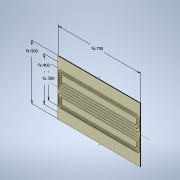
# Autodesk Inventor part: coil_layer_1R1
Saved by Autodesk Inventor 2021 (Build 250183000, 183)
## iProperties
Created: 2021-01-20
Part Number: coil_layer_1R1
Material: Generic
Document SubType Name: Modeling
Designer: phamv
Density: 1 g/cm^3
Appearance: Smooth - Ash
Author: phamv
Autodesk Inventor part; units mm, degrees
ref_plane "YZ Plane" through (0, 0, 0) normal (1, 0, 0) x (0, 1, 0)
ref_plane "XZ Plane" through (0, 0, 0) normal (0, 1, 0) x (-1, 0, 0)
ref_plane "XY Plane" through (0, 0, 0) normal (0, 0, 1) x (1, 0, 0)
sketch "layer_layout_sketch" plane through (0, 0, 0) normal (0, 0, 1) x (1, 0, 0)
  line L0 (-375, 250) -> (375, 250)
  line L1 (375, 250) -> (375, -250)
  line L2 (375, -250) -> (-375, -250)
  line L3 (-375, -250) -> (-375, 250)
  line L4 (0, 250) -> (0, -250) construction
  line L5 (-375, 200) -> (375, 200)
  line L6 (375, 200) -> (375, -200)
  line L7 (375, -200) -> (-375, -200)
  line L8 (-375, -200) -> (-375, 200)
  line L9 (0, 200) -> (0, -200) construction
  line L10 (-375, 150) -> (375, 150)
  line L11 (375, 150) -> (375, -150)
  line L12 (375, -150) -> (-375, -150)
  line L13 (-375, -150) -> (-375, 150)
  line L14 (0, 150) -> (0, -150) construction
  point P0 (0, 0)
  point P1 (0, 0)
  dimension "d116" = 500
  dimension "d117" = 750
  dimension "d122" = 400
  dimension "d123" = 300
  constraints: 30 end point, 9 midpoint, 6 parallel, 3 horizontal, 3 perpendicular, 2 collinear, 1 coincident, 1 vertical
  measures "d116" distance between parallel lines of L2 L0
  measures "d117" distance between parallel lines of L1 L3
  measures "d122" distance between parallel lines of L7 L5
  measures "d123" distance between parallel lines of L12 L10
sketch "coil_layer_sketch_lower" plane through (0, 0, 0) normal (0, 0, 1) x (1, 0, 0)
  line L0 (0, -9.3) -> (351.5, -9.3)
  line L1 (370, -27.8) -> (370, -131.5)
  line L2 (351.5, -150) -> (-351.5, -150)
  line L3 (-370, -131.5) -> (-370, -50.9)
  line L4 (0, -9.3) -> (0, -13.8)
  line L5 (0, -13.8) -> (350.5, -13.8)
  line L6 (365.5, -28.8) -> (365.5, -130.5)
  line L7 (350.5, -145.5) -> (-350.5, -145.5)
  line L8 (-351.5, -32.4) -> (338.75, -32.4)
  line L9 (357.25, -50.9) -> (357.25, -118.75)
  line L10 (338.75, -137.25) -> (-338.75, -137.25)
  line L11 (-365.5, -130.5) -> (-365.5, -51.9)
  line L12 (-350.5, -36.9) -> (337.75, -36.9)
  line L13 (352.75, -51.9) -> (352.75, -117.75)
  line L14 (337.75, -132.75) -> (-337.75, -132.75)
  line L15 (-352.75, -117.75) -> (-352.75, -75)
  line L16 (-357.25, -118.75) -> (-357.25, -74)
  line L17 (-338.75, -55.5) -> (326, -55.5)
  line L18 (344.5, -74) -> (344.5, -106)
  line L19 (-337.75, -60) -> (325, -60)
  line L20 (340, -75) -> (340, -105)
  line L21 (-523.3641, 0) -> (523.3641, 0) projected
  line L22 (325, -120) -> (-325, -120)
  line L23 (326, -124.5) -> (-326, -124.5)
  line L24 (-344.5, -106) -> (-344.5, -71.7563)
  line L25 (-344.5, -71.7563) -> (-340, -71.7563)
  line L26 (-340, -71.7563) -> (-340, -105)
  arc A0 (370, -27.8) -> (351.5, -9.3) centre (351.5, -27.8) ccw
  arc A1 (357.25, -50.9) -> (338.75, -32.4) centre (338.75, -50.9) ccw
  arc A2 (344.5, -74) -> (326, -55.5) centre (326, -74) ccw
  arc A3 (326, -124.5) -> (344.5, -106) centre (326, -106) ccw
  arc A4 (338.75, -137.25) -> (357.25, -118.75) centre (338.75, -118.75) ccw
  arc A5 (351.5, -150) -> (370, -131.5) centre (351.5, -131.5) ccw
  arc A6 (-370, -131.5) -> (-351.5, -150) centre (-351.5, -131.5) ccw
  arc A7 (-357.25, -118.75) -> (-338.75, -137.25) centre (-338.75, -118.75) ccw
  arc A8 (-344.5, -106) -> (-326, -124.5) centre (-326, -106) ccw
  arc A9 (-351.5, -32.4) -> (-370, -50.9) centre (-351.5, -50.9) ccw
  arc A10 (-338.75, -55.5) -> (-357.25, -74) centre (-338.75, -74) ccw
  arc A11 (-350.5, -36.9) -> (-365.5, -51.9) centre (-350.5, -51.9) ccw
  arc A12 (-337.75, -60) -> (-352.75, -75) centre (-337.75, -75) ccw
  arc A13 (-365.5, -130.5) -> (-350.5, -145.5) centre (-350.5, -130.5) ccw
  arc A14 (-352.75, -117.75) -> (-337.75, -132.75) centre (-337.75, -117.75) ccw
  arc A15 (-340, -105) -> (-325, -120) centre (-325, -105) ccw
  arc A16 (325, -120) -> (340, -105) centre (325, -105) ccw
  arc A17 (337.75, -132.75) -> (352.75, -117.75) centre (337.75, -117.75) ccw
  arc A18 (350.5, -145.5) -> (365.5, -130.5) centre (350.5, -130.5) ccw
  arc A19 (352.75, -51.9) -> (337.75, -36.9) centre (337.75, -51.9) ccw
  arc A20 (365.5, -28.8) -> (350.5, -13.8) centre (350.5, -28.8) ccw
  arc A21 (340, -75) -> (325, -60) centre (325, -75) ccw
  point P0 (0, 0)
  point P1 (0, 0)
  point P2 (368.0934, -60)
  point P3 (370, -61.9066)
  point P4 (0, -150)
  dimension "d1" = 4.5
  dimension "d2" = 4.5
  dimension "d3" = 4.5
  dimension "d4" = 9.3
  dimension "d5" = 740
  dimension "d6" = 370
  dimension "d7" = 4.5
  dimension "d8" = 4.5
  dimension "d9" = 8.25
  dimension "d10" = 4.5
  dimension "d11" = 18.6
  dimension "d12" = 4.5
  dimension "d13" = 8.25
  dimension "d14" = 4.5
  dimension "d15" = 4.5
  dimension "d16" = 4.5
  dimension "d17" = 8.25
  dimension "d19" = 18.6
  dimension "d20" = 8.25
  dimension "d82" = 150
  dimension "d88" = 4.5
  dimension "d89" = 8.25
  dimension "d96" = 4.5
  dimension "d97" = 8.25
  dimension "d98" = 18.5
  dimension "d99" = 15
  dimension "d109" = 15
  constraints: 52 end point, 44 point on circle, 44 tangent, 22 centre point, 19 equal radius, 15 perpendicular, 4 horizontal, 4 vertical, 3 parallel, 1 coincident, 1 midpoint
  measures "d1" distance between parallel lines of L5 L0
  measures "d2" distance between parallel lines of L6 L1
  measures "d3" distance between parallel lines of L2 L7
  measures "d4" distance from line of L21 L0.start
  measures "d5" distance between parallel lines of L3 L1
  measures "d6" distance from line of point (0, 0) L1
  measures "d7" distance between parallel lines of L3 L11
  measures "d8" distance between parallel lines of L13 L9
  measures "d9" distance between parallel lines of L9 L6
  measures "d10" distance between parallel lines of L8 L12
  measures "d11" distance between parallel lines of L8 L5
  measures "d12" distance between parallel lines of L10 L14
  measures "d13" distance between parallel lines of L7 L10
  measures "d14" distance between parallel lines of L16 L15
  measures "d15" distance between parallel lines of L17 L19
  measures "d16" distance between parallel lines of L20 L18
  measures "d17" distance between parallel lines of L18 L13
  measures "d19" distance between parallel lines of L17 L12
  measures "d20" distance between parallel lines of L11 L16
  measures "d82" distance between parallel lines of L2 L21
  measures "d88" distance between parallel lines of L23 L22
  measures "d89" distance between parallel lines of L14 L23
  measures "d96" distance between parallel lines of L24 L26
  measures "d97" distance between parallel lines of L15 L24
  measures "d98" radius of A0
  measures "d99" radius of A11
  measures "d109" radius of A21
sketch "coil_layer_sketch_upper" plane through (0, 0, 0) normal (0, 0, 1) x (1, 0, 0)
  line L0 (0, -13.8) -> (-351.5, -13.8)
  line L1 (-370, 4.7) -> (-370, 131.5)
  line L2 (-351.5, 150) -> (351.5, 150)
  line L3 (370, 131.5) -> (370, 27.8)
  line L4 (0, -9.3) -> (-350.5, -9.3)
  line L5 (-365.5, 5.7) -> (-365.5, 130.5)
  line L6 (-350.5, 145.5) -> (350.5, 145.5)
  line L7 (365.5, 130.5) -> (365.5, 28.8)
  line L8 (350.5, 13.8) -> (-337.75, 13.8)
  line L9 (-352.75, 28.8) -> (-352.75, 117.75)
  line L10 (351.5, 9.3) -> (-338.75, 9.3)
  line L11 (-357.25, 27.8) -> (-357.25, 118.75)
  line L12 (-337.75, 132.75) -> (337.75, 132.75)
  line L13 (-338.75, 137.25) -> (338.75, 137.25)
  line L14 (352.75, 117.75) -> (352.75, 51.9)
  line L15 (337.75, 36.9) -> (-325, 36.9)
  line L16 (357.25, 118.75) -> (357.25, 50.9)
  line L17 (338.75, 32.4) -> (-326, 32.4)
  line L18 (-340, 51.9) -> (-340, 105)
  line L19 (-325, 120) -> (325, 120)
  line L20 (340, 105) -> (340, 75)
  line L21 (325, 60) -> (-331.75, 60)
  line L22 (-344.5, 50.9) -> (-344.5, 106)
  line L23 (-326, 124.5) -> (326, 124.5)
  line L24 (344.5, 106) -> (344.5, 74)
  line L25 (326, 55.5) -> (-331.75, 55.5)
  line L26 (-331.75, 60) -> (-331.75, 55.5)
  line L27 (-700, 0) -> (700, 0)
  line L28 (-980, 0) -> (980, 0) projected
  line L29 (0, -13.8) -> (0, -9.3)
  line L30 (0, -51.9241) -> (0, 188.1241) projected
  arc A0 (340, 105) -> (325, 120) centre (325, 105) ccw
  arc A1 (325, 60) -> (340, 75) centre (325, 75) ccw
  arc A2 (352.75, 117.75) -> (337.75, 132.75) centre (337.75, 117.75) ccw
  arc A3 (337.75, 36.9) -> (352.75, 51.9) centre (337.75, 51.9) ccw
  arc A4 (365.5, 130.5) -> (350.5, 145.5) centre (350.5, 130.5) ccw
  arc A5 (350.5, 13.8) -> (365.5, 28.8) centre (350.5, 28.8) ccw
  arc A6 (-325, 120) -> (-340, 105) centre (-325, 105) ccw
  arc A7 (-340, 51.9) -> (-325, 36.9) centre (-325, 51.9) ccw
  arc A8 (-352.75, 28.8) -> (-337.75, 13.8) centre (-337.75, 28.8) ccw
  arc A9 (-365.5, 5.7) -> (-350.5, -9.3) centre (-350.5, 5.7) ccw
  arc A10 (-337.75, 132.75) -> (-352.75, 117.75) centre (-337.75, 117.75) ccw
  arc A11 (-350.5, 145.5) -> (-365.5, 130.5) centre (-350.5, 130.5) ccw
  arc A12 (-351.5, 150) -> (-370, 131.5) centre (-351.5, 131.5) ccw
  arc A13 (-338.75, 137.25) -> (-357.25, 118.75) centre (-338.75, 118.75) ccw
  arc A14 (-326, 124.5) -> (-344.5, 106) centre (-326, 106) ccw
  arc A15 (-344.5, 50.9) -> (-326, 32.4) centre (-326, 50.9) ccw
  arc A16 (-357.25, 27.8) -> (-338.75, 9.3) centre (-338.75, 27.8) ccw
  arc A17 (-370, 4.7) -> (-351.5, -13.8) centre (-351.5, 4.7) ccw
  arc A18 (326, 55.5) -> (344.5, 74) centre (326, 74) ccw
  arc A19 (338.75, 32.4) -> (357.25, 50.9) centre (338.75, 50.9) ccw
  arc A20 (351.5, 9.3) -> (370, 27.8) centre (351.5, 27.8) ccw
  arc A21 (370, 131.5) -> (351.5, 150) centre (351.5, 131.5) ccw
  arc A22 (357.25, 118.75) -> (338.75, 137.25) centre (338.75, 118.75) ccw
  arc A23 (344.5, 106) -> (326, 124.5) centre (326, 106) ccw
  point P0 (0, 0)
  point P1 (370, 9.3)
  point P2 (-357.25, 9.3)
  point P3 (0, 150)
  point P4 (-700, 0)
  point P5 (700, 0)
  point P6 (0, 150)
  dimension "d58" = 4.5
  dimension "d59" = 4.5
  dimension "d60" = 4.5
  dimension "d61" = 8.25
  dimension "d62" = 8.25
  dimension "d64" = 4.5
  dimension "d65" = 4.5
  dimension "d66" = 4.5
  dimension "d67" = 8.25
  dimension "d69" = 18.6
  dimension "d70" = 4.5
  dimension "d71" = 4.5
  dimension "d72" = 18.6
  dimension "d73" = 8.25
  dimension "d74" = 8.25
  dimension "d75" = 4.5
  dimension "d77" = 18.6
  dimension "d78" = 4.5
  dimension "d79" = 4.5
  dimension "d80" = 4.5
  dimension "d83" = 150
  dimension "d87" = 8.25
  dimension "d91" = 4.5
  dimension "d92" = 9.3
  dimension "d93" = 740
  dimension "d100" = 15
  dimension "d101" = 18.5
  dimension "d102" = 8.25
  constraints: 56 end point, 48 point on circle, 48 tangent, 24 centre point, 22 equal radius, 16 perpendicular, 5 point on line, 4 horizontal, 4 parallel, 3 vertical, 1 coincident, 1 collinear, 1 midpoint, 3 other
  measures "d58" distance between parallel lines of L1 L5
  measures "d59" distance between parallel lines of L2 L6
  measures "d60" distance between parallel lines of L7 L3
  measures "d61" distance between parallel lines of L13 L6
  measures "d62" distance between parallel lines of L5 L11
  measures "d64" distance between parallel lines of L10 L8
  measures "d65" distance between parallel lines of L14 L16
  measures "d66" distance between parallel lines of L13 L12
  measures "d67" distance between parallel lines of L16 L7
  measures "d69" distance between parallel lines of L4 L10
  measures "d70" distance between parallel lines of L11 L9
  measures "d71" distance between parallel lines of L17 L15
  measures "d72" distance between parallel lines of L8 L17
  measures "d73" distance between parallel lines of L12 L23
  measures "d74" distance between parallel lines of L9 L22
  measures "d75" distance between parallel lines of L23 L19
  measures "d77" distance between parallel lines of L15 L25
  measures "d78" distance between parallel lines of L24 L20
  measures "d79" distance between parallel lines of L25 L21
  measures "d80" distance between parallel lines of L22 L18
  measures "d83" distance of the line from the sketch origin of L2
  measures "d87" distance between parallel lines of L18 L26
  measures "d91" distance between parallel lines of L0 L4
  measures "d92" distance between parallel lines of L28 L4
  measures "d93" distance between parallel lines of L3 L1
  measures "d100" radius of A0
  measures "d101" radius of A12
  measures "d102" distance between parallel lines of L14 L24
extrude "layer_sheet Extrude" add sketch "layer_layout_sketch" along normal blind 4.5
extrude "wire_holes_upper Cut" cut sketch "coil_layer_sketch_upper" along normal blind 4.5 contours L0 A17 L27 A9 L4 L29 | A17 L1 A12 L2 L30 L6 A11 L5 A9 L27 | L30 L8 A5 L7 A4 L6 L2 A21 L3 A20 L10 | L10 A16 L11 A13 L13 L30 L12 A10 L9 A8 L8 | L30 L15 A3 L14 A2 L12 L13 A22 L16 A19 L17 | L17 A15 L22 A14 L23 L30 L19 A6 L18 A7 L15 | L30 L21 A1 L20 A0 L19 L23 A23 L24 A18 L25 | L25 L26 L21 L30
extrude "wire_holes_lower Cut" cut sketch "coil_layer_sketch_lower" along normal blind 4.5
equation "\"d1\" = wire_diameter"
equation "\"d2\" = wire_diameter"
equation "\"d3\" = wire_diameter"
equation "\"d4\" = 0.5 * distance_between_wires"
equation "\"d6\" = 0.5 * coil_length"
equation "\"d7\" = wire_diameter"
equation "\"d8\" = wire_diameter"
equation "\"d9\" = distance_between_wires_edge"
equation "\"d10\" = wire_diameter"
equation "\"d11\" = distance_between_wires"
equation "\"d12\" = wire_diameter"
equation "\"d13\" = distance_between_wires_edge"
equation "\"d14\" = wire_diameter"
equation "\"d15\" = wire_diameter"
equation "\"d16\" = wire_diameter"
equation "\"d17\" = distance_between_wires_edge"
equation "\"d19\" = distance_between_wires"
equation "\"d20\" = distance_between_wires_edge"
equation "\"d82\" = 0.5 * track_width"
equation "\"d58\" = wire_diameter"
equation "\"d59\" = wire_diameter"
equation "\"d60\" = wire_diameter"
equation "\"d61\" = distance_between_wires_edge"
equation "\"d62\" = distance_between_wires_edge"
equation "\"d64\" = wire_diameter"
equation "\"d65\" = wire_diameter"
equation "\"d66\" = wire_diameter"
equation "\"d67\" = distance_between_wires_edge"
equation "\"d69\" = distance_between_wires"
equation "\"d70\" = wire_diameter"
equation "\"d71\" = wire_diameter"
equation "\"d72\" = distance_between_wires"
equation "\"d73\" = distance_between_wires_edge"
equation "\"d74\" = distance_between_wires_edge"
equation "\"d75\" = wire_diameter"
equation "\"d77\" = distance_between_wires"
equation "\"d78\" = wire_diameter"
equation "\"d79\" = wire_diameter"
equation "\"d80\" = wire_diameter"
equation "\"d83\" = 0.5 * track_width"
equation "\"wire_diameter\" = 4.5"
equation "\"distance_between_wires\" = -1.2 * wire_diameter + 0.2 * parameter_6"
equation "\"distance_between_wires_edge\" = 8.25"
equation "\"bend_radius_inner\" = 15"
equation "\"bend_radius_outer\" = 18.5"
equation "\"ferrite_length\" = 109"
equation "\"ferrite_width\" = 15"
equation "\"ferrite_height\" = 8"
equation "\"edge_gap_distance\" = 14.5"
equation "\"parameter_5\" = 117.66667"
equation "\"bolt_diameter\" = 8"
equation "\"y_offset_for_bolts\" = 175"
equation "\"wall_thickness\" = 25"
equation "\"track_width\" = 300"
equation "\"parameter_6\" = 120"
equation "\"coil_length\" = 740"
body "Solid6"
